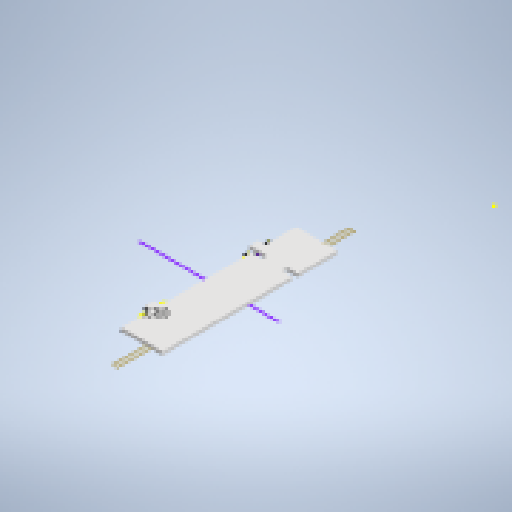
# Autodesk Inventor part: крепление Y
Saved by Autodesk Inventor 2024.2 (Build 282272000, 272)
## iProperties
Created: 2026-02-01
Part Number: крепление Y
Material: Типовые
Document SubType Name: Modeling
Designer: katya_notebook
Density: 1 g/cm^3
Appearance: По умолчанию
Author: katya_notebook
Autodesk Inventor part; units mm, degrees
ref_plane "YZ Plane" through (0, 0, 0) normal (1, 0, 0) x (0, 1, 0)
ref_plane "XZ Plane" through (0, 0, 0) normal (0, 1, 0) x (-1, 0, 0)
ref_plane "XY Plane" through (0, 0, 0) normal (0, 0, 1) x (1, 0, 0)
ref_plane "РабПлоскость1" through (-53.4845, 288.2505, 354.5129) normal (0, 1, 0) x (-1, 0, 0)
sketch "Эскиз1" plane through (-53.4845, 288.2505, 354.5129) normal (0, 1, 0) x (-1, 0, 0)
  line L0 (32.7, -62.75) -> (32.7, -56.5) projected
  line L1 (-13.3, 0) -> (-13.3, -240) projected
  line L2 (-13.3, -220) -> (32.7, -220)
  line L3 (32.7, -220) -> (32.7, -25)
  line L4 (32.7, -25) -> (-13.3, -25)
  line L5 (-13.3, -25) -> (-13.3, -220)
  line L6 (-5.3, -220) -> (142.8907, -220) projected
  line L7 (201.7, -25) -> (-5.3, -25) projected
  point P0 (-53.4845, -354.5129)
  point P1 (-13.3, -25)
  point P2 (-13.3, -220)
  dimension "d2" = 10
  dimension "d3" = 3.2
  constraints: 8 end point, 2 parallel, 2 point on line, 1 horizontal, 1 perpendicular
extrude "Выдавливание1" add sketch "Эскиз1" along normal blind 4
sketch "Эскиз2" plane through (-53.4845, 288.2505, 354.5129) normal (0, -1, 0) x (1, 0, 0)
  line L0 (-32.7, -165.5) -> (-32.7, -172.5) projected
  line L1 (-32.7, -165.5) -> (-38.7, -165.5) projected
  line L2 (-38.7, -172.5) -> (-38.7, -165.5) projected
  line L3 (-32.7, -172.5) -> (-38.7, -172.5) projected
  line L4 (-32.7, -188.5) -> (-32.7, -195.5) projected
  line L5 (-32.7, -188.5) -> (-38.7, -188.5) projected
  line L6 (-38.7, -195.5) -> (-38.7, -188.5) projected
  line L7 (-32.7, -195.5) -> (-38.7, -195.5) projected
  circle A0 centre (-35.7, -180.5) radius 1.75 projected
  line L8 (-37.8999, -64.576) -> (-32.1499, -64.576) projected
  circle A1 centre (-35.7, -64.5) radius 1.75 projected
  line L9 (-38.7, -79.5) -> (-38.7, -72.5) projected
  line L10 (-32.7, -72.5) -> (-32.7, -79.5) projected
  line L11 (-38.7, -56.5) -> (-38.7, -49.5) projected
  line L12 (-32.8499, -56.124) -> (-32.8499, -45.124) projected
  line L13 (-32.7, -49.5) -> (-38.7, -49.5) projected
  line L14 (-32.7, -220) -> (-32.7, -25) projected
  line L15 (-32.7, -59.324) -> (-30.2517, -59.324)
  line L16 (-30.2517, -59.324) -> (-30.2517, -69.324)
  line L17 (-30.2517, -69.324) -> (-32.7, -69.324)
  line L18 (-32.7, -69.324) -> (-32.7, -59.324)
  line L19 (-111.002, -122.5) -> (45.2006, -122.5)
  line L20 (-37.8999, -180.424) -> (-32.1499, -180.424)
  circle A2 centre (-35.7, -180.5) radius 1.75
  line L21 (-38.7, -165.5) -> (-38.7, -172.5)
  line L22 (-32.7, -172.5) -> (-32.7, -165.5)
  line L23 (-38.7, -188.5) -> (-38.7, -195.5)
  line L24 (-32.8499, -188.876) -> (-32.8499, -199.876)
  line L25 (-32.7, -195.5) -> (-38.7, -195.5)
  line L26 (-32.7, -25) -> (-32.7, -220)
  line L27 (-32.7, -185.676) -> (-30.2517, -185.676)
  line L28 (-30.2517, -185.676) -> (-30.2517, -175.676)
  line L29 (-30.2517, -175.676) -> (-32.7, -175.676)
  line L30 (-32.7, -175.676) -> (-32.7, -185.676)
  point P0 (53.4845, -354.5129)
  dimension "d2" = 10
  dimension "d3" = 3.2
  constraints: 32 end point, 11 symmetric about line, 2 horizontal, 2 parallel, 1 centre point, 1 perpendicular, 1 point on line, 4 other
  measures "d2" distance of L15.end L16.end
  measures "d3" vertical distance of L15.start L12.start
sketch "Эскиз3" plane through (-86.1845, 288.2505, 134.5129) normal (-1, 0, 0) x (0, 0, 1)
  line L0 (0, 0) -> (195, 0) projected
  line L1 (0, 4) -> (195, 4) projected
  line L2 (44.3461, 0) -> (34.3461, 0)
  line L3 (34.3461, 0) -> (34.3461, 4)
  line L4 (34.3461, 4) -> (44.3461, 4)
  line L5 (44.3461, 4) -> (44.3461, 0)
  line L6 (160.6836, 0) -> (150.6836, 0)
  line L7 (150.6836, 0) -> (150.6836, 4)
  line L8 (150.6836, 4) -> (160.6836, 4)
  line L9 (160.6836, 4) -> (160.6836, 0)
  point P0 (-134.5129, -288.2505)
  point P1 (44.3461, 4)
  point P2 (34.3461, 0)
  point P3 (160.6836, 4)
  point P4 (150.6836, 0)
  dimension "d4" = 10
  dimension "d5" = 10
  constraints: 16 end point, 4 parallel, 4 point on line, 2 horizontal, 2 perpendicular
  measures "d4" distance of L3.end L4.end
  measures "d5" distance of L7.end L8.end
extrude "Выдавливание2" add sketch "Эскиз3" along normal blind 8 contours L3 L1 L5 L0 | L7 L1 L9 L0
sketch "Эскиз4" plane through (-53.4845, 288.2505, 354.5129) normal (0, -1, 0) x (1, 0, 0)
  point P0 (53.4845, -354.5129)
  dimension "d2" = 10
  dimension "d3" = 3.2
sketch "Эскиз5" plane through (-53.4845, 288.2505, 354.5129) normal (0, -1, 0) x (1, 0, 0)
  point P0 (53.4845, -354.5129)
  dimension "d2" = 10
  dimension "d3" = 3.2
sketch "Эскиз6" plane through (-53.4845, 288.2505, 354.5129) normal (0, -1, 0) x (1, 0, 0)
  line L0 (-32.7, -175.6539) -> (-32.7, -69.3164) projected
  line L1 (-32.7, -175.6539) -> (-20.7, -175.6539)
  line L2 (-20.7, -175.6539) -> (-20.7, -169.6539)
  line L3 (-20.7, -169.6539) -> (-32.7, -169.6539)
  line L4 (-32.7, -169.6539) -> (-32.7, -175.6539)
  line L5 (13.3, -25) -> (13.3, -220) projected
  line L6 (13.3, -175.6539) -> (1.3, -175.6539)
  line L7 (1.3, -175.6539) -> (1.3, -169.6539)
  line L8 (1.3, -169.6539) -> (13.3, -169.6539)
  line L9 (13.3, -169.6539) -> (13.3, -175.6539)
  line L10 (-32.7, -219.9852) -> (-32.7, -25)
  line L11 (-32.7, -219.9852) -> (-32.7, -122.4926)
  line L12 (-32.7, -122.4852) -> (37.5594, -122.4852)
  line L13 (-32.7, -69.3164) -> (-20.7, -69.3164)
  line L14 (-20.7, -69.3164) -> (-20.7, -75.3164)
  line L15 (-20.7, -75.3164) -> (-32.7, -75.3164)
  line L16 (-32.7, -75.3164) -> (-32.7, -69.3164)
  line L17 (13.3, -69.3164) -> (1.3, -69.3164)
  line L18 (1.3, -69.3164) -> (1.3, -75.3164)
  line L19 (1.3, -75.3164) -> (13.3, -75.3164)
  line L20 (13.3, -75.3164) -> (13.3, -69.3164)
  point P0 (53.4845, -354.5129)
  point P1 (13.3, -169.6539)
  point P2 (-32.7, -169.6539)
  point P3 (13.3, -75.3164)
  point P4 (13.3, -69.3164)
  dimension "d2" = 10
  dimension "d3" = 3.2
  dimension "d8" = 6
  dimension "d9" = 12
  dimension "d12" = 97.5
  constraints: 38 end point, 7 symmetric about line, 6 point on line, 4 parallel, 3 horizontal, 2 midpoint, 2 perpendicular, 1 collinear, 1 vertical
  measures "d8" distance of L1.end L2.end
  measures "d9" distance of L2.end L3.end
  measures "d12" distance of L10.start L12.start
extrude "Выдавливание3" cut sketch "Эскиз6" against normal blind 8
sketch "Эскиз7" plane through (-53.4845, 288.2505, 354.5129) normal (0, -1, 0) x (1, 0, 0)
  line L0 (-12.95, -175.6539) -> (-12.95, -169.6539) projected
  line L1 (-7.95, -169.6539) -> (-7.95, -175.6539) projected
  line L2 (-6.45, -175.6539) -> (-6.45, -169.6539) projected
  line L3 (-11.45, -175.6539) -> (-11.45, -169.6539) projected
  line L4 (-12.95, -175.6539) -> (-12.95, -169.6539) projected
  line L5 (-11.45, -175.6539) -> (-7.95, -175.6539)
  line L6 (-7.95, -175.6539) -> (-7.95, -169.6539)
  line L7 (-7.95, -169.6539) -> (-11.45, -169.6539)
  line L8 (-11.45, -169.6539) -> (-11.45, -175.6539)
  circle A0 centre (-9.7, -172.6539) radius 1.75
  line L9 (-32.7, -169.6539) -> (-32.7, -75.3164) projected
  line L10 (-32.7, -122.4852) -> (36.9657, -122.4852)
  line L11 (-12.95, -69.3164) -> (-12.95, -75.3164)
  line L12 (-7.95, -75.3164) -> (-7.95, -69.3164)
  line L13 (-6.45, -69.3164) -> (-6.45, -75.3164)
  line L14 (-11.45, -69.3164) -> (-11.45, -75.3164)
  line L15 (-12.95, -69.3164) -> (-12.95, -75.3164)
  line L16 (-11.45, -69.3164) -> (-7.95, -69.3164)
  line L17 (-7.95, -69.3164) -> (-7.95, -75.3164)
  line L18 (-7.95, -75.3164) -> (-11.45, -75.3164)
  line L19 (-11.45, -75.3164) -> (-11.45, -69.3164)
  circle A1 centre (-9.7, -72.3164) radius 1.75
  point P0 (53.4845, -354.5129)
  dimension "d2" = 10
  dimension "d3" = 3.2
  constraints: 28 end point, 11 symmetric about line, 2 centre point, 2 horizontal, 2 parallel, 1 midpoint, 1 perpendicular, 1 tangent, 1 other
extrude "Выдавливание4" cut sketch "Эскиз7" against normal blind 8 contours A0 | A1
